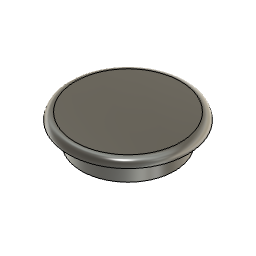
Amazon wheel cap (Autodesk Fusion 360 design; units mm, degrees)
Autodesk Fusion 360 part; units mm, degrees
sketch "Skizze1" plane through (0, 0, 0) normal (0, 0, 1) x (1, 0, 0)
  circle A0 centre (0, 0) radius 13.25
  dimension "d1" = 26.5
  constraint coincident A0.centre origin
  measures "d1" diameter of A0
extrude "Extrusion1" add sketch "Skizze1" along normal blind 6
sketch "Skizze2" plane through (0, 0, 6) normal (0, 0, 1) x (-1, 0, 0)
  circle A0 centre (0, 0) radius 13.25
  circle A1 centre (0, 0) radius 17
  dimension "d4" = 34
  constraint concentric A0 A1
  measures "d4" diameter of A1
extrude "Extrusion2" add sketch "Skizze2" along normal blind 2 contours A0 | A1
fillet "Abrundung1" radius 2 1 edges at (15.8496, 6.1475, 8)
